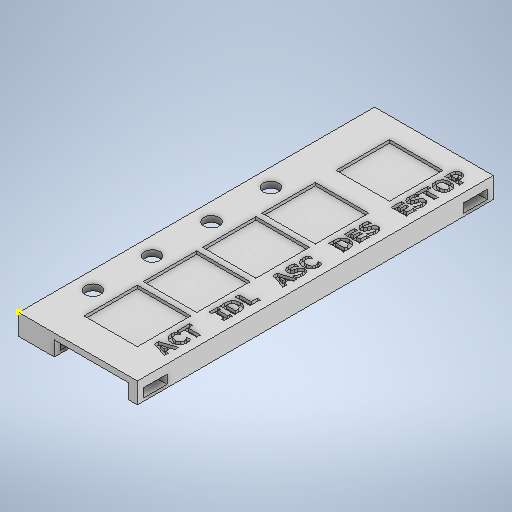
# Autodesk Inventor part: backpackstrap
Saved by Autodesk Inventor 2025.2 (Build 292293000, 293)
## iProperties
Created: 2025-01-16
Part Number: backpackstrap
Material: Generic
Document SubType Name: Modeling
Designer: email
Density: 1 g/cm^3
Appearance: Default
Author: email
Autodesk Inventor part; units mm, degrees
ref_plane "YZ Plane" through (0, 0, 0) normal (1, 0, 0) x (0, 1, 0)
ref_plane "XZ Plane" through (0, 0, 0) normal (0, 1, 0) x (-1, 0, 0)
ref_plane "XY Plane" through (0, 0, 0) normal (0, 0, 1) x (1, 0, 0)
sketch "Sketch1" plane through (0, 0, 0) normal (0, 1, 0) x (-1, 0, 0)
  line L0 (0, 0) -> (-40, 0)
  line L1 (-40, 0) -> (-40, -120)
  line L2 (-40, -120) -> (0, -120)
  line L3 (0, -120) -> (0, 0)
  line L4 (-30, -10) -> (-12, -10)
  line L5 (-12, -10) -> (-12, -28)
  line L6 (-12, -28) -> (-30, -28)
  line L7 (-30, -28) -> (-30, -10)
  line L8 (-12, -48) -> (-30, -48)
  line L9 (-30, -48) -> (-30, -30)
  line L10 (-12, -30) -> (-12, -48)
  line L11 (-30, -30) -> (-12, -30)
  line L12 (-12, -68) -> (-30, -68)
  line L13 (-30, -68) -> (-30, -50)
  line L14 (-12, -50) -> (-12, -68)
  line L15 (-30, -50) -> (-12, -50)
  line L16 (-12, -88) -> (-30, -88)
  line L17 (-30, -88) -> (-30, -70)
  line L18 (-12, -70) -> (-12, -88)
  line L19 (-30, -70) -> (-12, -70)
  circle A0 centre (-6, -19) radius 2.6
  circle A1 centre (-6, -39) radius 2.6
  circle A2 centre (-6, -59) radius 2.6
  circle A3 centre (-6, -79) radius 2.6
  line L20 (-12, -95) -> (-30, -95)
  line L21 (-30, -95) -> (-30, -113)
  line L22 (-30, -113) -> (-12, -113)
  line L23 (-12, -113) -> (-12, -95)
  point P0 (-30, -19)
  point P1 (-21, -10)
  point P2 (-30, -39)
  point P3 (-21, -30)
  point P4 (-30, -59)
  point P5 (-21, -50)
  point P6 (-30, -79)
  point P7 (-21, -70)
  point P8 (-12, -19)
  dimension "d0" = 120
  dimension "d1" = 40
  dimension "d2" = 18
  dimension "d3" = 18
  dimension "d4" = 10
  dimension "d5" = 10
  dimension "d8" = 20
  dimension "d14" = 6
  dimension "d16" = 19
  dimension "d17" = 5.2
  dimension "d20" = 20
  dimension "d72" = 7
  dimension "d73" = 18
  dimension "d74" = 18
  dimension "d75" = 7
  constraints: 48 end point, 6 parallel, 4 centre point, 3 horizontal, 3 midpoint, 3 perpendicular, 2 vertical, 36 other
  measures "d0" distance of L0.end L1.end
  measures "d1" distance of L0.start L0.end
  measures "d2" distance of L6.end L4.start
  measures "d3" distance of L4.start L4.end
  measures "d4" distance from line of L1 point (-30, -19)
  measures "d5" distance from line of L0 point (-21, -10)
  measures "d8" distance of L5.end L8.start
  measures "d14" distance of point (-12, -19) A0.centre
  measures "d16" distance from line of L0 A0.centre
  measures "d17" diameter of A0
  measures "d20" distance of A0.centre A1.centre
  measures "d72" distance between parallel lines of L16 L20
  measures "d73" distance of L22.end L20.start
  measures "d74" distance of L20.start L20.end
  measures "d75" distance between parallel lines of L2 L22
extrude "Extrusion1" add sketch "Sketch1" along normal blind 7
extrude "Extrusion4" add sketch "Sketch1" along normal blind 6 contours L4 L5 L6 L7 | L8 L9 L11 L10 | L12 L13 L15 L14 | L16 L17 L19 L18 | L23 L22 L21 L20
sketch "Sketch2" plane through (0, 0, 0) normal (0, -1, 0) x (1, 0, 0)
  line L0 (40, -120) -> (0, -120) projected
  line L1 (37, 0) -> (12, 0)
  line L2 (12, 0) -> (12, -120)
  line L3 (12, -120) -> (37, -120)
  line L4 (37, -120) -> (37, 0)
  line L5 (40, 0) -> (40, -120) projected
  line L6 (16.7261, -11.4981) -> (-4.7261, -11.4981)
  line L7 (-4.7261, -11.4981) -> (-4.7261, -26.5019)
  line L8 (-4.7261, -26.5019) -> (16.7261, -26.5019)
  line L9 (16.7261, -26.5019) -> (16.7261, -11.4981)
  line L10 (16.7261, -11.4981) -> (-4.7261, -26.5019) construction
  line L11 (-4.7261, -11.4981) -> (16.7261, -26.5019) construction
  line L12 (16.7261, -31.4981) -> (-4.7261, -31.4981)
  line L13 (-4.7261, -31.4981) -> (-4.7261, -46.5019)
  line L14 (-4.7261, -46.5019) -> (16.7261, -46.5019)
  line L15 (16.7261, -46.5019) -> (16.7261, -31.4981)
  line L16 (16.7261, -31.4981) -> (-4.7261, -46.5019) construction
  line L17 (-4.7261, -31.4981) -> (16.7261, -46.5019) construction
  line L18 (16.7261, -51.4981) -> (-4.7261, -51.4981)
  line L19 (-4.7261, -51.4981) -> (-4.7261, -66.5019)
  line L20 (-4.7261, -66.5019) -> (16.7261, -66.5019)
  line L21 (16.7261, -66.5019) -> (16.7261, -51.4981)
  line L22 (16.7261, -51.4981) -> (-4.7261, -66.5019) construction
  line L23 (-4.7261, -51.4981) -> (16.7261, -66.5019) construction
  line L24 (16.7261, -71.4981) -> (-4.7261, -71.4981)
  line L25 (-4.7261, -71.4981) -> (-4.7261, -86.5019)
  line L26 (-4.7261, -86.5019) -> (16.7261, -86.5019)
  line L27 (16.7261, -86.5019) -> (16.7261, -71.4981)
  line L28 (16.7261, -71.4981) -> (-4.7261, -86.5019) construction
  line L29 (-4.7261, -71.4981) -> (16.7261, -86.5019) construction
  point P0 (0, 0)
  point P1 (12, -5.4474)
  point P2 (12, -22.1252)
  point P3 (6, -19)
  point P4 (12, -42.1252)
  point P5 (6, -39)
  point P6 (12, -62.1252)
  point P7 (6, -59)
  point P8 (12, -82.1252)
  point P9 (6, -79)
  point P10 (12, -26.5019)
  point P11 (12, -11.4981)
  point P12 (12, -46.5019)
  point P13 (12, -31.4981)
  point P14 (12, -66.5019)
  point P15 (12, -51.4981)
  point P16 (12, -86.5019)
  point P17 (12, -71.4981)
  dimension "d27" = 25
  dimension "d28" = 3
  dimension "d40" = 20
  constraints: 56 end point, 4 parallel, 3 point on line, 2 horizontal, 2 midpoint, 2 perpendicular, 1 vertical, 36 other
  measures "d27" distance between parallel lines of L2 L4
  measures "d28" distance between parallel lines of L5 L4
  measures "d40" distance of point (12, -22.125) point (12, -42.125)
extrude "Extrusion2" cut sketch "Sketch2" against normal blind 5
sketch "Sketch3" plane through (40, 0, 0) normal (1, 0, 0) x (0, 0, -1)
  line L0 (2, 4) -> (10, 4)
  line L1 (10, 4) -> (10, 1)
  line L2 (10, 1) -> (2, 1)
  line L3 (2, 1) -> (2, 4)
  line L4 (0, 0) -> (120, 0) projected
  line L5 (0, 0) -> (0, 7) projected
  line L6 (118, 1) -> (110, 1)
  line L7 (110, 1) -> (110, 4)
  line L8 (110, 4) -> (118, 4)
  line L9 (118, 4) -> (118, 1)
  line L10 (120, 0) -> (120, 7) projected
  dimension "d45" = 8
  dimension "d46" = 3
  dimension "d47" = 1
  dimension "d48" = 2
  dimension "d49" = 2
  dimension "d50" = 1
  dimension "d51" = 8
  dimension "d52" = 3
  constraints: 16 end point, 4 parallel, 2 horizontal, 2 perpendicular
  measures "d45" distance of L0.start L0.end
  measures "d46" distance of L2.end L0.start
  measures "d47" distance between parallel lines of L4 L2
  measures "d48" distance between parallel lines of L5 L3
  measures "d49" distance between parallel lines of L10 L9
  measures "d50" distance between parallel lines of L4 L6
  measures "d51" distance of L7.end L8.end
  measures "d52" distance of L6.end L7.end
extrude "Extrusion3" cut sketch "Sketch3" against normal through all
sketch "Sketch4" plane through (0, 7, 0) normal (0, 1, 0) x (1, 0, 0)
  point P0 (0, 0)
sketch "Sketch5" plane through (0, 7, 0) normal (0, 1, 0) x (1, 0, 0)
  line L0 (32, 12) -> (32, 26) construction
  line L1 (32, 26) -> (28.7488, 26) construction
  line L2 (28.7488, 26) -> (28.7488, 12) construction
  line L3 (28.7488, 12) -> (32, 12) construction
  line L4 (30, 10) -> (12, 10) projected
  line L5 (32, 32) -> (32, 46) construction
  line L6 (32, 46) -> (28.5985, 46) construction
  line L7 (28.5985, 46) -> (28.5985, 32) construction
  line L8 (28.5985, 32) -> (32, 32) construction
  line L9 (32, 52) -> (32, 66) construction
  line L10 (32, 66) -> (28.2667, 66) construction
  line L11 (28.2667, 66) -> (28.2667, 52) construction
  line L12 (28.2667, 52) -> (32, 52) construction
  line L13 (32, 72) -> (32, 86) construction
  line L14 (32, 86) -> (28.2667, 86) construction
  line L15 (28.2667, 86) -> (28.2667, 72) construction
  line L16 (28.2667, 72) -> (32, 72) construction
  line L17 (30, 30) -> (12, 30) projected
  line L18 (30, 28) -> (30, 10) projected
  line L19 (30, 48) -> (30, 30) projected
  line L20 (30, 68) -> (30, 50) projected
  line L21 (30, 88) -> (30, 70) projected
  line L22 (30, 50) -> (12, 50) projected
  line L23 (30, 70) -> (12, 70) projected
  line L24 (28.9568, 93) -> (32, 93) construction
  line L25 (32, 93) -> (32, 107) construction
  line L26 (32, 107) -> (28.9568, 107) construction
  line L27 (28.9568, 107) -> (28.9568, 93) construction
  line L28 (40, 120) -> (0, 120) projected
  line L29 (30, 113) -> (30, 95) projected
  line L30 (37.0972, 11.9797) -> (32.0972, 13.6694)
  line L31 (32.0972, 13.6694) -> (32.0972, 15.0389)
  line L32 (32.0972, 15.0389) -> (37.0972, 16.7285)
  line L33 (37.0972, 16.7285) -> (37.0972, 15.436)
  line L34 (37.0972, 15.436) -> (36.0762, 15.124)
  line L35 (36.0762, 15.124) -> (36.0762, 13.5519)
  line L36 (36.0762, 13.5519) -> (37.0972, 13.2358)
  line L37 (37.0972, 13.2358) -> (37.0972, 11.9797)
  line L38 (35.1686, 14.8485) -> (33.5154, 14.3379)
  line L39 (33.5154, 14.3379) -> (35.1686, 13.8233)
  line L40 (35.1686, 13.8233) -> (35.1686, 14.8485)
  spline S0 degree 2 poles (37.1945, 19.3825) (37.1945, 18.2561) (35.8331, 16.9352) (34.6013, 16.9352) knots 0 0 0 1 2 2 2
  spline S1 degree 2 poles (34.6013, 16.9352) (33.4141, 16.9352) (32, 18.2601) (32, 19.3865) knots 0 0 0 1 2 2 2
  spline S2 degree 2 poles (32, 19.3865) (32, 19.6823) (32.0689, 20.1605) (32.1256, 20.3793) knots 0 0 0 1 2 2 2
  spline S3 degree 2 poles (32.1256, 20.3793) (32.1783, 20.5494) (32.3525, 20.9506) (32.4173, 21.0762) knots 0 0 0 1 2 2 2
  line L41 (32.4173, 21.0762) -> (33.6086, 21.0762)
  line L42 (33.6086, 21.0762) -> (33.6086, 20.9506)
  spline S4 degree 2 poles (33.6086, 20.9506) (33.5276, 20.8574) (33.3006, 20.5818) (33.1953, 20.4076) knots 0 0 0 1 2 2 2
  spline S5 degree 2 poles (33.1953, 20.4076) (33.0859, 20.2334) (32.936, 19.816) (32.936, 19.5851) knots 0 0 0 1 2 2 2
  spline S6 degree 2 poles (32.936, 19.5851) (32.936, 19.3136) (33.1062, 18.8639) (33.3209, 18.6572) knots 0 0 0 1 2 2 2
  spline S7 degree 2 poles (33.3209, 18.6572) (33.5113, 18.4708) (34.1637, 18.2318) (34.6053, 18.2318) knots 0 0 0 1 2 2 2
  spline S8 degree 2 poles (34.6053, 18.2318) (35.0713, 18.2318) (35.7075, 18.4789) (35.9019, 18.6815) knots 0 0 0 1 2 2 2
  spline S9 degree 2 poles (35.9019, 18.6815) (36.0924, 18.876) (36.2585, 19.3541) (36.2585, 19.5932) knots 0 0 0 1 2 2 2
  spline S10 degree 2 poles (36.2585, 19.5932) (36.2585, 19.8404) (36.0924, 20.2901) (35.9911, 20.4441) knots 0 0 0 1 2 2 2
  spline S11 degree 2 poles (35.9911, 20.4441) (35.8898, 20.6143) (35.675, 20.8695) (35.59, 20.9627) knots 0 0 0 1 2 2 2
  line L43 (35.59, 20.9627) -> (35.59, 21.0762)
  line L44 (35.59, 21.0762) -> (36.765, 21.0762)
  spline S12 degree 2 poles (36.765, 21.0762) (36.8298, 20.9384) (36.9919, 20.5778) (37.0486, 20.3833) knots 0 0 0 1 2 2 2
  spline S13 degree 2 poles (37.0486, 20.3833) (37.1216, 20.1483) (37.1945, 19.7391) (37.1945, 19.3825) knots 0 0 0 1 2 2 2
  line L45 (37.0972, 22.778) -> (33.0494, 22.778)
  line L46 (33.0494, 22.778) -> (33.0494, 21.299)
  line L47 (33.0494, 21.299) -> (32.0972, 21.299)
  line L48 (32.0972, 21.299) -> (32.0972, 25.513)
  line L49 (32.0972, 25.513) -> (33.0494, 25.513)
  line L50 (33.0494, 25.513) -> (33.0494, 24.034)
  line L51 (33.0494, 24.034) -> (37.0972, 24.034)
  line L52 (37.0972, 24.034) -> (37.0972, 22.778)
  line L53 (37, 35.0065) -> (37, 32.316)
  line L54 (37, 32.316) -> (36.1288, 32.316)
  line L55 (36.1288, 32.316) -> (36.1288, 33.0332)
  line L56 (36.1288, 33.0332) -> (32.8712, 33.0332)
  line L57 (32.8712, 33.0332) -> (32.8712, 32.316)
  line L58 (32.8712, 32.316) -> (32, 32.316)
  line L59 (32, 32.316) -> (32, 35.0065)
  line L60 (32, 35.0065) -> (32.8712, 35.0065)
  line L61 (32.8712, 35.0065) -> (32.8712, 34.2893)
  line L62 (32.8712, 34.2893) -> (36.1288, 34.2893)
  line L63 (36.1288, 34.2893) -> (36.1288, 35.0065)
  line L64 (36.1288, 35.0065) -> (37, 35.0065)
  spline S14 degree 2 poles (34.5041, 40.3023) (35.205, 40.3023) (36.3071, 39.6904) (36.6029, 39.2245) knots 0 0 0 1 2 2 2
  spline S15 degree 2 poles (36.6029, 39.2245) (36.8541, 38.8355) (37, 37.9198) (37, 37.4052) knots 0 0 0 1 2 2 2
  line L65 (37, 37.4052) -> (37, 35.8412)
  line L66 (37, 35.8412) -> (32, 35.8412)
  line L67 (32, 35.8412) -> (32, 37.389)
  spline S16 degree 2 poles (32, 37.389) (32, 37.9157) (32.1337, 38.8355) (32.393, 39.2407) knots 0 0 0 1 2 2 2
  spline S17 degree 2 poles (32.393, 39.2407) (32.7091, 39.731) (33.7788, 40.3023) (34.5041, 40.3023) knots 0 0 0 1 2 2 2
  spline S18 degree 2 poles (34.4959, 39.0138) (34.0016, 39.0138) (33.2966, 38.6734) (33.0981, 38.325) knots 0 0 0 1 2 2 2
  spline S19 degree 2 poles (33.0981, 38.325) (32.9603, 38.0697) (32.9319, 37.5105) (32.9319, 37.1216) knots 0 0 0 1 2 2 2
  line L68 (32.9319, 37.1216) -> (32.9319, 37.0972)
  line L69 (32.9319, 37.0972) -> (36.064, 37.0972)
  line L70 (36.064, 37.0972) -> (36.064, 37.1216)
  spline S20 degree 2 poles (36.064, 37.1216) (36.064, 37.5429) (36.0357, 38.1224) (35.8695, 38.3857) knots 0 0 0 1 2 2 2
  spline S21 degree 2 poles (35.8695, 38.3857) (35.675, 38.6937) (34.9903, 39.0138) (34.4959, 39.0138) knots 0 0 0 1 2 2 2
  line L71 (37, 44.3825) -> (37, 41.0478)
  line L72 (37, 41.0478) -> (32, 41.0478)
  line L73 (32, 41.0478) -> (32, 42.3039)
  line L74 (32, 42.3039) -> (36.0478, 42.3039)
  line L75 (36.0478, 42.3039) -> (36.0478, 44.3825)
  line L76 (36.0478, 44.3825) -> (37, 44.3825)
  line L77 (37.0972, 51.9797) -> (32.0972, 53.6694)
  line L78 (32.0972, 53.6694) -> (32.0972, 55.0389)
  line L79 (32.0972, 55.0389) -> (37.0972, 56.7285)
  line L80 (37.0972, 56.7285) -> (37.0972, 55.436)
  line L81 (37.0972, 55.436) -> (36.0762, 55.124)
  line L82 (36.0762, 55.124) -> (36.0762, 53.5519)
  line L83 (36.0762, 53.5519) -> (37.0972, 53.2358)
  line L84 (37.0972, 53.2358) -> (37.0972, 51.9797)
  line L85 (35.1686, 54.8485) -> (33.5154, 54.3379)
  line L86 (33.5154, 54.3379) -> (35.1686, 53.8233)
  line L87 (35.1686, 53.8233) -> (35.1686, 54.8485)
  spline S22 degree 2 poles (37.1864, 58.7707) (37.1864, 58.1953) (36.9635, 57.3282) (36.8015, 56.9554) knots 0 0 0 1 2 2 2
  line L88 (36.8015, 56.9554) -> (35.6102, 56.9554)
  line L89 (35.6102, 56.9554) -> (35.6102, 57.0689)
  spline S23 degree 2 poles (35.6102, 57.0689) (35.9303, 57.4457) (36.2747, 58.3493) (36.2747, 58.7747) knots 0 0 0 1 2 2 2
  spline S24 degree 2 poles (36.2747, 58.7747) (36.2747, 58.8841) (36.2261, 59.2366) (36.1775, 59.342) knots 0 0 0 1 2 2 2
  spline S25 degree 2 poles (36.1775, 59.342) (36.1207, 59.4716) (35.9141, 59.654) (35.748, 59.654) knots 0 0 0 1 2 2 2
  spline S26 degree 2 poles (35.748, 59.654) (35.5575, 59.654) (35.3225, 59.3582) (35.2699, 59.1556) knots 0 0 0 1 2 2 2
  spline S27 degree 2 poles (35.2699, 59.1556) (35.201, 58.9003) (35.0835, 58.3209) (34.9943, 58.0656) knots 0 0 0 1 2 2 2
  spline S28 degree 2 poles (34.9943, 58.0656) (34.7917, 57.4862) (34.0989, 56.9838) (33.5802, 56.9838) knots 0 0 0 1 2 2 2
  spline S29 degree 2 poles (33.5802, 56.9838) (32.8793, 56.9838) (32.0081, 58.171) (32.0081, 59.0624) knots 0 0 0 1 2 2 2
  spline S30 degree 2 poles (32.0081, 59.0624) (32.0081, 59.5081) (32.1904, 60.3914) (32.3444, 60.7399) knots 0 0 0 1 2 2 2
  line L90 (32.3444, 60.7399) -> (33.487, 60.7399)
  line L91 (33.487, 60.7399) -> (33.487, 60.6305)
  spline S31 degree 2 poles (33.487, 60.6305) (33.248, 60.3509) (32.9198, 59.5486) (32.9198, 59.1272) knots 0 0 0 1 2 2 2
  spline S32 degree 2 poles (32.9198, 59.1272) (32.9198, 58.9611) (32.9684, 58.7018) (33.0332, 58.5559) knots 0 0 0 1 2 2 2
  spline S33 degree 2 poles (33.0332, 58.5559) (33.0859, 58.4384) (33.2966, 58.2682) (33.4263, 58.2682) knots 0 0 0 1 2 2 2
  spline S34 degree 2 poles (33.4263, 58.2682) (33.6207, 58.2682) (33.8436, 58.5397) (33.9327, 58.9287) knots 0 0 0 1 2 2 2
  spline S35 degree 2 poles (33.9327, 58.9287) (33.9895, 59.1799) (34.0989, 59.6459) (34.1921, 59.9133) knots 0 0 0 1 2 2 2
  spline S36 degree 2 poles (34.1921, 59.9133) (34.3825, 60.4319) (35.0146, 60.9384) (35.5332, 60.9384) knots 0 0 0 1 2 2 2
  spline S37 degree 2 poles (35.5332, 60.9384) (36.2788, 60.9384) (37.1864, 59.7674) (37.1864, 58.7707) knots 0 0 0 1 2 2 2
  spline S38 degree 2 poles (37.1945, 63.7382) (37.1945, 62.6118) (35.8331, 61.2909) (34.6013, 61.2909) knots 0 0 0 1 2 2 2
  spline S39 degree 2 poles (34.6013, 61.2909) (33.4141, 61.2909) (32, 62.6159) (32, 63.7423) knots 0 0 0 1 2 2 2
  spline S40 degree 2 poles (32, 63.7423) (32, 64.0381) (32.0689, 64.5162) (32.1256, 64.735) knots 0 0 0 1 2 2 2
  spline S41 degree 2 poles (32.1256, 64.735) (32.1783, 64.9052) (32.3525, 65.3063) (32.4173, 65.4319) knots 0 0 0 1 2 2 2
  line L92 (32.4173, 65.4319) -> (33.6086, 65.4319)
  line L93 (33.6086, 65.4319) -> (33.6086, 65.3063)
  spline S42 degree 2 poles (33.6086, 65.3063) (33.5276, 65.2131) (33.3006, 64.9376) (33.1953, 64.7634) knots 0 0 0 1 2 2 2
  spline S43 degree 2 poles (33.1953, 64.7634) (33.0859, 64.5891) (32.936, 64.1718) (32.936, 63.9408) knots 0 0 0 1 2 2 2
  spline S44 degree 2 poles (32.936, 63.9408) (32.936, 63.6694) (33.1062, 63.2196) (33.3209, 63.013) knots 0 0 0 1 2 2 2
  spline S45 degree 2 poles (33.3209, 63.013) (33.5113, 62.8266) (34.1637, 62.5875) (34.6053, 62.5875) knots 0 0 0 1 2 2 2
  spline S46 degree 2 poles (34.6053, 62.5875) (35.0713, 62.5875) (35.7075, 62.8347) (35.9019, 63.0373) knots 0 0 0 1 2 2 2
  spline S47 degree 2 poles (35.9019, 63.0373) (36.0924, 63.2318) (36.2585, 63.7099) (36.2585, 63.9489) knots 0 0 0 1 2 2 2
  spline S48 degree 2 poles (36.2585, 63.9489) (36.2585, 64.1961) (36.0924, 64.6459) (35.9911, 64.7998) knots 0 0 0 1 2 2 2
  spline S49 degree 2 poles (35.9911, 64.7998) (35.8898, 64.97) (35.675, 65.2253) (35.59, 65.3185) knots 0 0 0 1 2 2 2
  line L94 (35.59, 65.3185) -> (35.59, 65.4319)
  line L95 (35.59, 65.4319) -> (36.765, 65.4319)
  spline S50 degree 2 poles (36.765, 65.4319) (36.8298, 65.2942) (36.9919, 64.9335) (37.0486, 64.7391) knots 0 0 0 1 2 2 2
  spline S51 degree 2 poles (37.0486, 64.7391) (37.1216, 64.5041) (37.1945, 64.0948) (37.1945, 63.7382) knots 0 0 0 1 2 2 2
  spline S52 degree 2 poles (34.5932, 76.9797) (35.2942, 76.9797) (36.3963, 76.3679) (36.6921, 75.9019) knots 0 0 0 1 2 2 2
  spline S53 degree 2 poles (36.6921, 75.9019) (36.9433, 75.513) (37.0891, 74.5972) (37.0891, 74.0827) knots 0 0 0 1 2 2 2
  line L96 (37.0891, 74.0827) -> (37.0891, 72.5186)
  line L97 (37.0891, 72.5186) -> (32.0891, 72.5186)
  line L98 (32.0891, 72.5186) -> (32.0891, 74.0665)
  spline S54 degree 2 poles (32.0891, 74.0665) (32.0891, 74.5932) (32.2229, 75.513) (32.4822, 75.9182) knots 0 0 0 1 2 2 2
  spline S55 degree 2 poles (32.4822, 75.9182) (32.7982, 76.4084) (33.8679, 76.9797) (34.5932, 76.9797) knots 0 0 0 1 2 2 2
  spline S56 degree 2 poles (34.5851, 75.6912) (34.0908, 75.6912) (33.3857, 75.3509) (33.1872, 75.0024) knots 0 0 0 1 2 2 2
  spline S57 degree 2 poles (33.1872, 75.0024) (33.0494, 74.7472) (33.0211, 74.188) (33.0211, 73.799) knots 0 0 0 1 2 2 2
  line L99 (33.0211, 73.799) -> (33.0211, 73.7747)
  line L100 (33.0211, 73.7747) -> (36.1532, 73.7747)
  line L101 (36.1532, 73.7747) -> (36.1532, 73.799)
  spline S58 degree 2 poles (36.1532, 73.799) (36.1532, 74.2204) (36.1248, 74.7998) (35.9587, 75.0632) knots 0 0 0 1 2 2 2
  spline S59 degree 2 poles (35.9587, 75.0632) (35.7642, 75.3712) (35.0794, 75.6912) (34.5851, 75.6912) knots 0 0 0 1 2 2 2
  line L102 (37.0891, 77.7253) -> (32.0891, 77.7253)
  line L103 (32.0891, 77.7253) -> (32.0891, 81.1045)
  line L104 (32.0891, 81.1045) -> (33.0413, 81.1045)
  line L105 (33.0413, 81.1045) -> (33.0413, 78.9733)
  line L106 (33.0413, 78.9733) -> (33.9206, 78.9733)
  line L107 (33.9206, 78.9733) -> (33.9206, 80.9384)
  line L108 (33.9206, 80.9384) -> (34.8728, 80.9384)
  line L109 (34.8728, 80.9384) -> (34.8728, 78.9733)
  line L110 (34.8728, 78.9733) -> (36.137, 78.9733)
  line L111 (36.137, 78.9733) -> (36.137, 81.1045)
  line L112 (36.137, 81.1045) -> (37.0891, 81.1045)
  line L113 (37.0891, 81.1045) -> (37.0891, 77.7253)
  spline S60 degree 2 poles (37.1783, 83.4992) (37.1783, 82.9238) (36.9554, 82.0567) (36.7934, 81.684) knots 0 0 0 1 2 2 2
  line L114 (36.7934, 81.684) -> (35.6021, 81.684)
  line L115 (35.6021, 81.684) -> (35.6021, 81.7974)
  spline S61 degree 2 poles (35.6021, 81.7974) (35.9222, 82.1742) (36.2666, 83.0778) (36.2666, 83.5032) knots 0 0 0 1 2 2 2
  spline S62 degree 2 poles (36.2666, 83.5032) (36.2666, 83.6126) (36.218, 83.9652) (36.1694, 84.0705) knots 0 0 0 1 2 2 2
  spline S63 degree 2 poles (36.1694, 84.0705) (36.1126, 84.2002) (35.906, 84.3825) (35.7399, 84.3825) knots 0 0 0 1 2 2 2
  spline S64 degree 2 poles (35.7399, 84.3825) (35.5494, 84.3825) (35.3144, 84.0867) (35.2618, 83.8841) knots 0 0 0 1 2 2 2
  spline S65 degree 2 poles (35.2618, 83.8841) (35.1929, 83.6288) (35.0754, 83.0494) (34.9862, 82.7942) knots 0 0 0 1 2 2 2
  spline S66 degree 2 poles (34.9862, 82.7942) (34.7836, 82.2147) (34.0908, 81.7123) (33.5721, 81.7123) knots 0 0 0 1 2 2 2
  spline S67 degree 2 poles (33.5721, 81.7123) (32.8712, 81.7123) (32, 82.8995) (32, 83.7909) knots 0 0 0 1 2 2 2
  spline S68 degree 2 poles (32, 83.7909) (32, 84.2366) (32.1823, 85.1199) (32.3363, 85.4684) knots 0 0 0 1 2 2 2
  line L116 (32.3363, 85.4684) -> (33.4789, 85.4684)
  line L117 (33.4789, 85.4684) -> (33.4789, 85.359)
  spline S69 degree 2 poles (33.4789, 85.359) (33.2399, 85.0794) (32.9117, 84.2771) (32.9117, 83.8558) knots 0 0 0 1 2 2 2
  spline S70 degree 2 poles (32.9117, 83.8558) (32.9117, 83.6896) (32.9603, 83.4303) (33.0251, 83.2844) knots 0 0 0 1 2 2 2
  spline S71 degree 2 poles (33.0251, 83.2844) (33.0778, 83.1669) (33.2885, 82.9968) (33.4182, 82.9968) knots 0 0 0 1 2 2 2
  spline S72 degree 2 poles (33.4182, 82.9968) (33.6126, 82.9968) (33.8355, 83.2682) (33.9246, 83.6572) knots 0 0 0 1 2 2 2
  spline S73 degree 2 poles (33.9246, 83.6572) (33.9814, 83.9084) (34.0908, 84.3744) (34.184, 84.6418) knots 0 0 0 1 2 2 2
  spline S74 degree 2 poles (34.184, 84.6418) (34.3744, 85.1605) (35.0065, 85.6669) (35.5251, 85.6669) knots 0 0 0 1 2 2 2
  spline S75 degree 2 poles (35.5251, 85.6669) (36.2707, 85.6669) (37.1783, 84.4959) (37.1783, 83.4992) knots 0 0 0 1 2 2 2
  line L118 (37.1053, 93.5186) -> (32.1053, 93.5186)
  line L119 (32.1053, 93.5186) -> (32.1053, 96.8979)
  line L120 (32.1053, 96.8979) -> (33.0575, 96.8979)
  line L121 (33.0575, 96.8979) -> (33.0575, 94.7666)
  line L122 (33.0575, 94.7666) -> (33.9368, 94.7666)
  line L123 (33.9368, 94.7666) -> (33.9368, 96.7318)
  line L124 (33.9368, 96.7318) -> (34.889, 96.7318)
  line L125 (34.889, 96.7318) -> (34.889, 94.7666)
  line L126 (34.889, 94.7666) -> (36.1532, 94.7666)
  line L127 (36.1532, 94.7666) -> (36.1532, 96.8979)
  line L128 (36.1532, 96.8979) -> (37.1053, 96.8979)
  line L129 (37.1053, 96.8979) -> (37.1053, 93.5186)
  spline S76 degree 2 poles (37.1945, 99.2925) (37.1945, 98.7172) (36.9716, 97.8501) (36.8096, 97.4773) knots 0 0 0 1 2 2 2
  line L130 (36.8096, 97.4773) -> (35.6183, 97.4773)
  line L131 (35.6183, 97.4773) -> (35.6183, 97.5908)
  spline S77 degree 2 poles (35.6183, 97.5908) (35.9384, 97.9676) (36.2828, 98.8712) (36.2828, 99.2966) knots 0 0 0 1 2 2 2
  spline S78 degree 2 poles (36.2828, 99.2966) (36.2828, 99.406) (36.2342, 99.7585) (36.1856, 99.8639) knots 0 0 0 1 2 2 2
  spline S79 degree 2 poles (36.1856, 99.8639) (36.1288, 99.9935) (35.9222, 100.1759) (35.7561, 100.1759) knots 0 0 0 1 2 2 2
  spline S80 degree 2 poles (35.7561, 100.1759) (35.5656, 100.1759) (35.3306, 99.8801) (35.278, 99.6775) knots 0 0 0 1 2 2 2
  spline S81 degree 2 poles (35.278, 99.6775) (35.2091, 99.4222) (35.0916, 98.8428) (35.0024, 98.5875) knots 0 0 0 1 2 2 2
  spline S82 degree 2 poles (35.0024, 98.5875) (34.7998, 98.0081) (34.107, 97.5057) (33.5883, 97.5057) knots 0 0 0 1 2 2 2
  spline S83 degree 2 poles (33.5883, 97.5057) (32.8874, 97.5057) (32.0162, 98.6929) (32.0162, 99.5843) knots 0 0 0 1 2 2 2
  spline S84 degree 2 poles (32.0162, 99.5843) (32.0162, 100.03) (32.1985, 100.9133) (32.3525, 101.2618) knots 0 0 0 1 2 2 2
  line L132 (32.3525, 101.2618) -> (33.4951, 101.2618)
  line L133 (33.4951, 101.2618) -> (33.4951, 101.1524)
  spline S85 degree 2 poles (33.4951, 101.1524) (33.2561, 100.8728) (32.9279, 100.0705) (32.9279, 99.6491) knots 0 0 0 1 2 2 2
  spline S86 degree 2 poles (32.9279, 99.6491) (32.9279, 99.483) (32.9765, 99.2237) (33.0413, 99.0778) knots 0 0 0 1 2 2 2
  spline S87 degree 2 poles (33.0413, 99.0778) (33.094, 98.9603) (33.3047, 98.7901) (33.4344, 98.7901) knots 0 0 0 1 2 2 2
  spline S88 degree 2 poles (33.4344, 98.7901) (33.6288, 98.7901) (33.8517, 99.0616) (33.9408, 99.4506) knots 0 0 0 1 2 2 2
  spline S89 degree 2 poles (33.9408, 99.4506) (33.9976, 99.7018) (34.107, 100.1677) (34.2002, 100.4352) knots 0 0 0 1 2 2 2
  spline S90 degree 2 poles (34.2002, 100.4352) (34.3906, 100.9538) (35.0227, 101.4603) (35.5413, 101.4603) knots 0 0 0 1 2 2 2
  spline S91 degree 2 poles (35.5413, 101.4603) (36.2869, 101.4603) (37.1945, 100.2893) (37.1945, 99.2925) knots 0 0 0 1 2 2 2
  line L134 (37.1053, 103.0648) -> (33.0575, 103.0648)
  line L135 (33.0575, 103.0648) -> (33.0575, 101.5859)
  line L136 (33.0575, 101.5859) -> (32.1053, 101.5859)
  line L137 (32.1053, 101.5859) -> (32.1053, 105.7998)
  line L138 (32.1053, 105.7998) -> (33.0575, 105.7998)
  line L139 (33.0575, 105.7998) -> (33.0575, 104.3209)
  line L140 (33.0575, 104.3209) -> (37.1053, 104.3209)
  line L141 (37.1053, 104.3209) -> (37.1053, 103.0648)
  spline S92 degree 2 poles (34.6053, 110.8647) (35.8209, 110.8647) (37.2107, 109.5681) (37.2107, 108.4417) knots 0 0 0 1 2 2 2
  spline S93 degree 2 poles (37.2107, 108.4417) (37.2107, 107.3112) (35.8047, 106.0227) (34.6053, 106.0227) knots 0 0 0 1 2 2 2
  spline S94 degree 2 poles (34.6053, 106.0227) (33.4019, 106.0227) (32, 107.3112) (32, 108.4417) knots 0 0 0 1 2 2 2
  spline S95 degree 2 poles (32, 108.4417) (32, 109.5681) (33.3938, 110.8647) (34.6053, 110.8647) knots 0 0 0 1 2 2 2
  spline S96 degree 2 poles (34.6053, 109.5681) (34.1556, 109.5681) (33.5276, 109.3857) (33.329, 109.2277) knots 0 0 0 1 2 2 2
  spline S97 degree 2 poles (33.329, 109.2277) (33.1224, 109.0697) (32.9441, 108.6645) (32.9441, 108.4457) knots 0 0 0 1 2 2 2
  spline S98 degree 2 poles (32.9441, 108.4457) (32.9441, 108.2147) (33.1102, 107.8379) (33.3209, 107.6637) knots 0 0 0 1 2 2 2
  spline S99 degree 2 poles (33.3209, 107.6637) (33.5154, 107.5097) (34.1596, 107.3193) (34.6053, 107.3193) knots 0 0 0 1 2 2 2
  spline S100 degree 2 poles (34.6053, 107.3193) (35.0673, 107.3193) (35.675, 107.5016) (35.8817, 107.6596) knots 0 0 0 1 2 2 2
  spline S101 degree 2 poles (35.8817, 107.6596) (36.0883, 107.8177) (36.2666, 108.2269) (36.2666, 108.4457) knots 0 0 0 1 2 2 2
  spline S102 degree 2 poles (36.2666, 108.4457) (36.2666, 108.6686) (36.0762, 109.0818) (35.8736, 109.2318) knots 0 0 0 1 2 2 2
  spline S103 degree 2 poles (35.8736, 109.2318) (35.6548, 109.3938) (35.0754, 109.5681) (34.6053, 109.5681) knots 0 0 0 1 2 2 2
  spline S104 degree 2 poles (33.6815, 115.4554) (34.03, 115.4554) (34.6621, 115.2326) (34.8728, 115.0259) knots 0 0 0 1 2 2 2
  spline S105 degree 2 poles (34.8728, 115.0259) (35.0065, 114.9003) (35.2253, 114.5924) (35.3023, 114.41) knots 0 0 0 1 2 2 2
  spline S106 degree 2 poles (35.3023, 114.41) (35.3793, 114.2237) (35.4684, 113.7901) (35.4684, 113.5227) knots 0 0 0 1 2 2 2
  line L142 (35.4684, 113.5227) -> (35.4684, 112.8663)
  line L143 (35.4684, 112.8663) -> (37.1053, 112.8663)
  line L144 (37.1053, 112.8663) -> (37.1053, 111.6102)
  line L145 (37.1053, 111.6102) -> (32.1053, 111.6102)
  line L146 (32.1053, 111.6102) -> (32.1053, 113.5511)
  spline S107 degree 2 poles (32.1053, 113.5511) (32.1053, 113.9806) (32.2634, 114.6086) (32.4335, 114.8639) knots 0 0 0 1 2 2 2
  spline S108 degree 2 poles (32.4335, 114.8639) (32.624, 115.1475) (33.248, 115.4554) (33.6815, 115.4554) knots 0 0 0 1 2 2 2
  spline S109 degree 2 poles (33.7139, 114.1669) (33.4992, 114.1669) (33.1953, 113.9643) (33.1386, 113.8266) knots 0 0 0 1 2 2 2
  spline S110 degree 2 poles (33.1386, 113.8266) (33.0616, 113.6483) (33.0373, 113.3241) (33.0373, 113.0446) knots 0 0 0 1 2 2 2
  line L147 (33.0373, 113.0446) -> (33.0373, 112.8663)
  line L148 (33.0373, 112.8663) -> (34.5365, 112.8663)
  line L149 (34.5365, 112.8663) -> (34.5365, 112.9554)
  spline S111 degree 2 poles (34.5365, 112.9554) (34.5365, 113.1297) (34.5284, 113.4457) (34.5081, 113.5632) knots 0 0 0 1 2 2 2
  spline S112 degree 2 poles (34.5081, 113.5632) (34.4919, 113.6645) (34.3947, 113.8874) (34.3339, 113.9481) knots 0 0 0 1 2 2 2
  spline S113 degree 2 poles (34.3339, 113.9481) (34.2123, 114.0778) (33.9408, 114.1669) (33.7139, 114.1669) knots 0 0 0 1 2 2 2
  point P0 (0, 0)
  dimension "d57" = 14
  dimension "d58" = 2
  dimension "d59" = 14
  dimension "d60" = 14
  dimension "d61" = 14
  dimension "d62" = 2
  dimension "d63" = 2
  dimension "d64" = 2
  dimension "d65" = 2
  dimension "d66" = 2
  dimension "d67" = 2
  dimension "d68" = 2
  dimension "d69" = 14
  dimension "d76" = 13
  dimension "d77" = 2
  constraints: 10 other
  measures "d57" distance of L1.end L2.end
  measures "d58" distance between parallel lines of L4 L3
  measures "d59" distance of L6.end L8.start
  measures "d60" distance of L10.end L12.start
  measures "d61" distance of L14.end L16.start
  measures "d62" distance between parallel lines of L17 L8
  measures "d63" distance between parallel lines of L18 L0
  measures "d64" distance between parallel lines of L19 L5
  measures "d65" distance between parallel lines of L20 L9
  measures "d66" distance between parallel lines of L21 L13
  measures "d67" distance between parallel lines of L22 L12
  measures "d68" distance between parallel lines of L23 L16
  measures "d69" distance of L26.end L24.start
  measures "d76" distance between parallel lines of L28 L26
  measures "d77" distance between parallel lines of L29 L25
extrude "Extrusion5" cut sketch "Sketch5" against normal blind 1
body "Solid1"
